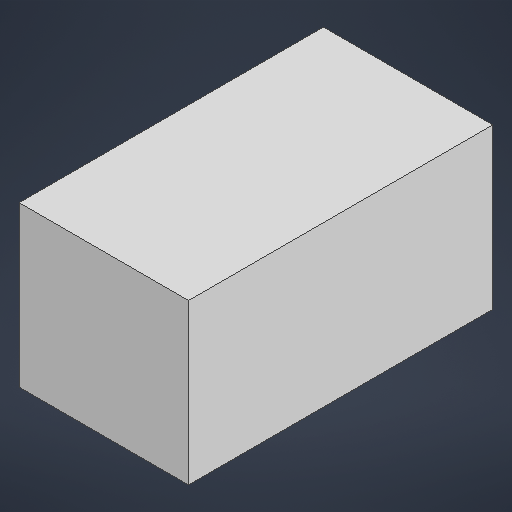
# Autodesk Inventor part: test
Saved by Autodesk Inventor 2026.1 (Build 301233000, 233)
## iProperties
Created: 2025-08-31
Part Number: test
Material: Generic
Document SubType Name: Modeling
Designer: junha
Density: 1 g/cm^3
Appearance: Default
Author: junha
Autodesk Inventor part; units mm, degrees
ref_plane "YZ Plane" through (0, 0, 0) normal (1, 0, 0) x (0, 1, 0)
ref_plane "XZ Plane" through (0, 0, 0) normal (0, 1, 0) x (-1, 0, 0)
ref_plane "XY Plane" through (0, 0, 0) normal (0, 0, 1) x (1, 0, 0)
sketch "Sketch1" plane through (0, 0, 0) normal (0, 1, 0) x (-1, 0, 0)
  line L0 (0, 0) -> (10.6062, 0)
  line L1 (10.6062, 0) -> (10.6062, -19.0483)
  line L2 (10.6062, -19.0483) -> (0, -19.0483)
  line L3 (0, -19.0483) -> (0, 0)
  constraints: 8 end point, 2 parallel, 1 horizontal, 1 perpendicular
extrude "Extrusion1" add sketch "Sketch1" along normal blind 10
body "Solid1"
